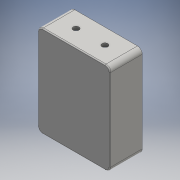
# Autodesk Inventor part: box_base
Saved by Autodesk Inventor 2016 (Build 200138000, 138)
## iProperties
Created: 2016-03-25
Part Number: box_base
Material: Generic
Document SubType Name: Modeling
Designer: Paschalis
Density: 1 g/cm^3
Appearance: Default
Author: Paschalis
Autodesk Inventor part; units mm, degrees
ref_plane "YZ Plane" through (0, 0, 0) normal (1, 0, 0) x (0, 1, 0)
ref_plane "XZ Plane" through (0, 0, 0) normal (0, 1, 0) x (-1, 0, 0)
ref_plane "XY Plane" through (0, 0, 0) normal (0, 0, 1) x (1, 0, 0)
sketch "Sketch1" plane through (0, 0, 0) normal (0, 1, 0) x (-1, 0, 0)
  line L0 (75, 95) -> (-75, 95)
  line L1 (-75, 95) -> (-75, -95)
  line L2 (-75, -95) -> (75, -95)
  line L3 (75, -95) -> (75, 95)
  point P0 (0, 0)
  point P1 (75, 0)
  point P2 (0, 95)
  dimension "d0" = 150
  dimension "d1" = 190
  constraints: 8 end point, 2 midpoint, 2 parallel, 1 horizontal, 1 horizontal alignment, 1 perpendicular, 1 vertical alignment
  measures "d0" distance of L2.end L1.end
  measures "d1" distance of L1.end L0.end
extrude "Extrusion1" add sketch "Sketch1" along normal blind 67
fillet "Fillet1" radius 10 4 edges at (75, 33.5, 95) (-75, 33.5, 95) (-75, 33.5, -95) (75, 33.5, -95)
sketch "Sketch2" plane through (0, 67, 0) normal (0, 1, 0) x (1, 0, 0)
  line L0 (-67.5, -88) -> (67.5, -88)
  line L1 (67.5, -88) -> (67.5, 88)
  line L2 (67.5, 88) -> (-67.5, 88)
  line L3 (-67.5, 88) -> (-67.5, -88)
  point P0 (0, 0)
  point P1 (0, -88)
  point P2 (-67.5, 0)
  dimension "d5" = 135
  dimension "d6" = 176
  constraints: 8 end point, 2 midpoint, 2 parallel, 1 horizontal, 1 horizontal alignment, 1 perpendicular, 1 vertical alignment
  measures "d5" distance of L2.end L1.end
  measures "d6" distance of L1.end L0.end
extrude "Extrusion2" cut sketch "Sketch2" against normal blind 62
fillet "Fillet2" radius 10 4 edges at (-67.5, 36, -88) (-67.5, 36, 88) (67.5, 36, -88) (67.5, 36, 88)
fillet "Fillet3" radius 2 8 edges at (72.0711, 0, -92.0711) (0, 0, -95) (-72.0711, 0, -92.0711) (-75, 0, 0) (-72.0711, 0, 92.0711) (0, 0, 95) (72.0711, 0, 92.0711) (75, 0, 0)
sketch "Sketch3" plane through (-65, 67, 95) normal (0, 0, 1) x (1, 0, 0)
  circle A0 centre (35, -32.5) radius 6
  circle A1 centre (95, -32.5) radius 6
  line L0 (35, -32.5) -> (95, -32.5) construction
  line L1 (-10, 0) -> (-10, -65) construction
  point P0 (65, -67)
  point P1 (65, -32.5)
  point P2 (-10, -32.5)
  dimension "d11" = 12
  dimension "d12" = 12
  dimension "d13" = 60
  constraints: 2 centre point, 2 end point, 2 midpoint, 1 horizontal, 1 horizontal alignment, 1 vertical alignment
  measures "d11" diameter of A0
  measures "d12" diameter of A1
  measures "d13" distance of L0.start L0.end
extrude "Extrusion3" cut sketch "Sketch3" against normal blind 200
body "Solid1"
